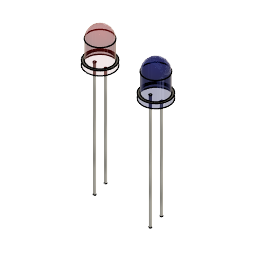
leds (Autodesk Fusion 360 design; units mm, degrees)
part number: 2026-03-28-21-06-32-198
Autodesk Fusion 360 part; units mm, degrees
sketch "Boceto1" plane through (0, 0, 0) normal (0, 0, 1) x (1, 0, 0)
  circle A0 centre (52.0206, 41.8833) radius 2.95
  circle A1 centre (-7, -7) radius 2.95
  circle A2 centre (-7, -7) radius 2.5
  line L0 (-9.95, -7.0073) -> (-9.5, -7.0073)
  dimension "d1" = 5.9
  dimension "d2" = 5.9
  dimension "d3" = 5
  dimension "d4" = 0.45
  constraint concentric A1 A2
  constraint coincident A1 L0.start
  constraint coincident A2 L0.end
  constraint horizontal L0
  measures "d1" diameter of A0
  measures "d2" diameter of A1
  measures "d3" diameter of A2
  measures "d4" distance of L0.start L0.end
extrude "Extruir1" add sketch "Boceto1" along normal blind 7.6 contours A2 makes body 1
extrude "Extruir2" add sketch "Boceto1" along normal blind 1 contours A1 bodies 1
fillet "Empalme1" radius 2.5 1 faces at (-6.1414, -6.4146, 7.6) on bodies 1
sketch "Boceto2" plane through (0, 0, 0) normal (0, 0, -1) x (1, 0, 0)
  circle A0 centre (-7, 7) radius 2.95
  line L0 (-9.5, 7) -> (-8.23, 7)
  circle A1 centre (-8.23, 7) radius 0.25
  line L1 (-4.5, 7) -> (-5.77, 7)
  circle A2 centre (-5.77, 7) radius 0.25
  dimension "d11" = 1.27
  dimension "d12" = 0.5
  dimension "d13" = 1.27
  dimension "d14" = 0.5
  constraint horizontal L0
  constraint coincident L0.end A1.centre
  constraint horizontal L1
  constraint coincident L1.end A2.centre
  measures "d11" distance of L0.start L0.end
  measures "d12" diameter of A1
  measures "d13" distance of L1.start L1.end
  measures "d14" diameter of A2
extrude "Extruir3" add sketch "Boceto2" along normal blind 25.4 contours A1 bodies 1
extrude "Extruir4" add sketch "Boceto2" along normal blind 22 contours A2 bodies 1
copy_body "CopiarPegarCuerpos1" bodies 1 makes body 2
move_body "Desplazar1" bodies 2 to x (1, 0, 0) y (0, 1, 0) z (0, 0, 1) at (12.4799, -0.1156, 0)
